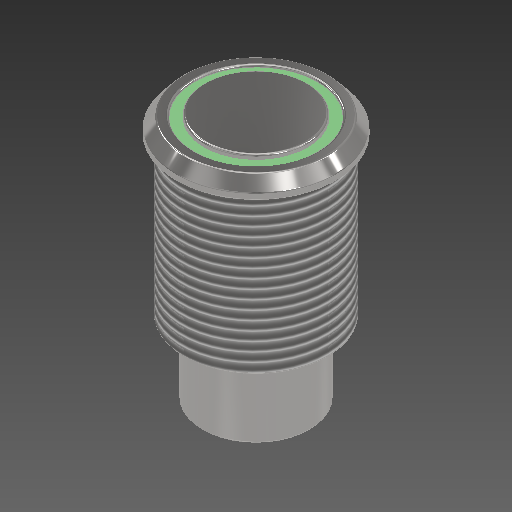
# Autodesk Inventor part: 16mm_momentary
Saved by Autodesk Inventor 2020.2 (Build 242310000, 310)
## iProperties
Created: 2020-04-11
Part Number: 16mm_momentary
Material: PVC-Piping
Document SubType Name: Modeling
Designer: agmlego
Mass: 6.81462 g
Surface Area: 17.4784 cm^2
Volume: 4.86759 cm^3
Density: 1.4 g/cm^3
Appearance: Steel - Polished
GlobalPropertyList: <PropertyList/>
Author: agmlego
Autodesk Inventor part; units mm, degrees
ref_plane "YZ Plane" through (0, 0, 0) normal (1, 0, 0) x (0, 1, 0)
ref_plane "XZ Plane" through (0, 0, 0) normal (0, 1, 0) x (-1, 0, 0)
ref_plane "XY Plane" through (0, 0, 0) normal (0, 0, 1) x (1, 0, 0)
sketch "Sketch1" plane through (0, 0, 0) normal (0, 0, 1) x (1, 0, 0)
  line L0 (0, 0) -> (0, 27.6)
  line L1 (0, 27.6) -> (5.75, 27.6)
  line L2 (8.9, 26.096) -> (8.9, 25.346)
  line L3 (8.9, 25.346) -> (8, 25.346)
  line L4 (8, 25.346) -> (8, 8)
  line L5 (8, 8) -> (6, 8)
  line L6 (6, 8) -> (6, 0)
  line L7 (6, 0) -> (0, 0)
  line L8 (5.75, 27.6) -> (5.75, 27.092)
  line L9 (5.75, 27.092) -> (6.8, 27.092)
  line L10 (6.8, 27.092) -> (6.8, 27.346)
  line L11 (6.8, 27.346) -> (7.85, 27.346)
  line L12 (7.85, 27.346) -> (8.9, 26.096)
  dimension "d0" = 8.9
  dimension "d1" = 5.75
  dimension "d2" = 6.8
  dimension "d3" = 0.254
  dimension "d4" = 0.254
  dimension "d5" = 2
  dimension "d6" = 8
  dimension "d7" = 6
  dimension "d9" = 27.6
  dimension "d10" = 8
  dimension "d11" = 0.75
  constraints: 26 end point, 9 perpendicular, 2 parallel, 2 vertical
  measures "d0" distance between parallel lines of L0 L2
  measures "d1" distance between parallel lines of L0 L8
  measures "d2" distance between parallel lines of L0 L10
  measures "d3" distance between parallel lines of L1 L11
  measures "d4" distance between parallel lines of L9 L11
  measures "d5" distance between parallel lines of L11 L3
  measures "d6" distance between parallel lines of L0 L4
  measures "d7" distance between parallel lines of L0 L6
  measures "d9" distance between parallel lines of L7 L1
  measures "d10" distance between parallel lines of L7 L5
  measures "d11" distance of L2.start L2.end
revolve "Revolution1" add sketch "Sketch1" angle 360 about axis through (0, 0, 0) along (0, 1, 0)
thread "Thread1" size "M16x1" class "6g" standard "ANSI Metric M Profile" full length
fillet "Fillet1" radius 0.25 7 edges at (-8.9, 26.096, 0) (-7.85, 27.346, 0) (-6.8, 27.346, 0) (-5.75, 27.6, 0) (-8.9, 25.346, 0) (-8, 8, 0) (-6, 0, 0)
sketch "Sketch2" plane through (0, 0, 0) normal (0, -1, 0) x (1, 0, 0)
  line L0 (0, -4.25) -> (0, 4.25) construction
  line L1 (-2.54, -2.54) -> (-2.54, 2.54) construction
  line L2 (-2.54, 0) -> (0, 0) construction
  dimension "d16" = 2.54
  dimension "d17" = 2.54
  dimension "d18" = 8.5
  constraints: 6 end point, 4 coincident, 2 midpoint, 1 horizontal, 1 perpendicular, 1 vertical
  measures "d16" distance of L2.start L2.end
  measures "d17" distance of L2.start L1.start
  measures "d18" distance of L0.start L0.end
body "Solid1"
